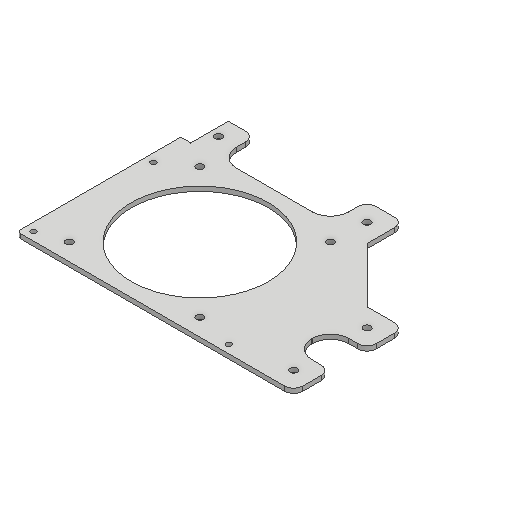
# Autodesk Inventor part: 3DP_PLA_Controller_Case_Top
Saved by Autodesk Inventor 2026.1 (Build 301233000, 233)
## iProperties
Created: 2017-05-26
Part Number: 3DP_PLA_Controller_Case_Top
Material: Ogólny
Document SubType Name: Modeling
Designer: Andrzej
Density: 1 g/cm^3
Appearance: Domyślna
Mass: 20.9942 g
Surface Area: 190.879 cm^2
Volume: 20.9942 cm^3
Author: Andrzej
Autodesk Inventor part; units mm, degrees
ref_plane "YZ Plane" through (0, 0, 0) normal (1, 0, 0) x (0, 1, 0)
ref_plane "XZ Plane" through (0, 0, 0) normal (0, 1, 0) x (-1, 0, 0)
ref_plane "XY Plane" through (0, 0, 0) normal (0, 0, 1) x (1, 0, 0)
sketch "Szkic1" plane through (0, 0, 0) normal (0, 0, 1) x (1, 0, 0)
  line L0 (0, 53.1646) -> (0, 0)
  line L1 (0, 0) -> (98.9175, 0)
  line L2 (98.9175, 0) -> (98.9175, 1.2597)
  line L3 (98.9175, 1.2597) -> (101.455, 3.8466)
  line L4 (101.455, 3.8466) -> (101.455, 38.0126)
  line L5 (101.455, 38.0126) -> (98.9175, 40.5017)
  line L6 (98.9175, 40.5017) -> (98.9175, 50.7051)
  line L7 (98.9175, 50.7051) -> (96.4101, 53.1646)
  line L8 (96.4101, 53.1646) -> (0, 53.1646)
  line L9 (-10, 93.1646) -> (141.455, 93.1646)
  line L10 (141.455, 93.1646) -> (141.455, -17)
  line L11 (141.455, -17) -> (-10, -17)
  line L12 (-10, -17) -> (-10, 93.1646)
  line L13 (91.455, 93.1646) -> (91.455, 43.1646)
  line L14 (91.455, 43.1646) -> (141.455, 43.1646)
  point P0 (-10, 13.9306)
  point P1 (7.9866, -17)
  dimension "d0" = 101.455
  dimension "d1" = 53.1646
  dimension "d2" = 98.9175
  dimension "d21" = 98.9175
  dimension "d22" = 1.2597
  dimension "d23" = 10.2034
  dimension "d24" = 34.166
  dimension "d33" = 40
  dimension "d34" = 40
  dimension "d35" = 17
  dimension "d36" = 10
  dimension "d37" = 50
  dimension "d38" = 50
  constraints: 30 end point, 4 point on line, 2 parallel, 2 perpendicular, 1 horizontal, 1 vertical
  measures "d0" distance between parallel lines of L4 L0
  measures "d1" distance between parallel lines of L1 L8
  measures "d2" distance between parallel lines of L0 L6
  measures "d21" distance between parallel lines of L0 L2
  measures "d22" distance of L2.start L2.end
  measures "d23" distance of L5.end L6.end
  measures "d24" distance of L3.end L5.start
  measures "d33" distance between parallel lines of L10 L4
  measures "d34" distance between parallel lines of L9 L8
  measures "d35" distance between parallel lines of L1 L11
  measures "d36" distance between parallel lines of L12 L0
  measures "d37" distance between parallel lines of L10 L13
  measures "d38" distance between parallel lines of L14 L9
extrude "Wyciągnięcie proste1" add sketch "Szkic1" along normal blind 2.5 contours L8 L13 L14 L6 L5 L4 L3 L2 L1 L0 | L0 L1 L2 L3 L4 L5 L6 L14 L10 L11 L12 L9 L13 L8
sketch "Szkic2" plane through (0, 0, 2.5) normal (0, 0, 1) x (1, 0, 0)
  line L0 (-10, 93.1646) -> (-10, -17) projected
  line L1 (-10, -17) -> (141.455, -17) projected
  line L2 (141.455, -17) -> (141.455, 43.1646) projected
  line L3 (141.455, 43.1646) -> (91.455, 43.1646) projected
  line L4 (91.455, 43.1646) -> (91.455, 93.1646) projected
  line L5 (91.455, 93.1646) -> (-10, 93.1646) projected
  line L6 (10, 93.1646) -> (10, 73.1646)
  line L7 (10, 73.1646) -> (71.455, 73.1646)
  line L8 (71.455, 73.1646) -> (71.455, 93.1646)
  line L9 (91.455, 93.1646) -> (-10, 93.1646) projected
  line L10 (141.455, -17) -> (141.455, 43.1646) projected
  line L11 (141.455, 23.1646) -> (121.455, 23.1646)
  line L12 (121.455, 23.1646) -> (121.455, 3)
  line L13 (121.455, 3) -> (141.455, 3)
  circle A0 centre (45, 28.0823) radius 37.5
  point P0 (0, 0)
  point P1 (131.455, -7)
  point P2 (131.455, 33.1646)
  point P3 (81.455, 83.1646)
  point P4 (0, 83.1646)
  point P5 (9.25, 63.8323)
  point P6 (80.75, 63.8323)
  point P7 (80.75, -7.6677)
  point P8 (9.25, -7.6677)
  dimension "d42" = 20
  dimension "d43" = 20
  dimension "d44" = 20
  dimension "d45" = 20
  dimension "d46" = 20
  dimension "d47" = 20
  dimension "d78" = 10
  dimension "d79" = 10
  dimension "d80" = 10
  dimension "d81" = 10
  dimension "d82" = 10
  dimension "d83" = 10
  dimension "d84" = 10
  dimension "d85" = 10
  dimension "d121" = 75
  dimension "d122" = 35.75
  dimension "d123" = 35.75
  dimension "d124" = 35.75
  dimension "d125" = 35.75
  dimension "d126" = 35.75
  dimension "d127" = 35.75
  dimension "d128" = 35.75
  dimension "d129" = 35.75
  dimension "d139" = 45.0823
  dimension "d140" = 101.455
  dimension "d141" = 90.1646
  dimension "d142" = 55
  constraints: 12 end point, 4 perpendicular, 4 point on line, 1 centre point, 1 horizontal, 1 vertical
  measures "d42" distance between parallel lines of L0 L6
  measures "d43" distance between parallel lines of L4 L8
  measures "d44" distance between parallel lines of L3 L11
  measures "d45" distance between parallel lines of L1 L13
  measures "d46" distance between parallel lines of L5 L7
  measures "d47" distance between parallel lines of L2 L12
  measures "d78" distance from line of L13 point (131.455, -7)
  measures "d79" distance from line of L3 point (131.455, 33.165)
  measures "d80" distance from line of L8 point (81.455, 83.165)
  measures "d81" distance from line of L6 point (0, 83.165)
  measures "d82" distance from line of L2 point (131.455, -7)
  measures "d83" distance from line of L2 point (131.455, 33.165)
  measures "d84" distance from line of L5 point (81.455, 83.165)
  measures "d85" distance from line of L9 point (0, 83.165)
  measures "d121" diameter of A0
  measures "d122" horizontal distance of point (9.25, 63.832) A0.centre
  measures "d123" horizontal distance of A0.centre point (9.25, 63.832)
  measures "d124" horizontal distance of A0.centre point (9.25, -7.668)
  measures "d125" horizontal distance of A0.centre point (9.25, -7.668)
  measures "d126" horizontal distance of point (80.75, 63.832) A0.centre
  measures "d127" horizontal distance of A0.centre point (80.75, 63.832)
  measures "d128" horizontal distance of A0.centre point (80.75, -7.668)
  measures "d129" horizontal distance of A0.centre point (80.75, -7.668)
  measures "d139" distance from line of L7 A0.centre
  measures "d140" distance between parallel lines of L0 L4
  measures "d141" distance between parallel lines of L1 L7
  measures "d142" distance from line of L0 A0.centre
fillet "Zaokrąglenie1" radius 5 4 edges at (-10, 93.1646, 1.25) (91.455, 93.1646, 1.25) (141.455, 43.1646, 1.25) (141.455, -17, 1.25)
hole "Otwór1" at (131.455, -7, 2.5) at (131.455, 33.1646, 2.5) at (81.455, 83.1646, 2.5) at (0, 83.1646, 2.5) direction (0, 0, -1) diameter 4 end through all
fillet "Zaokrąglenie2" radius 2 1 edges at (-10, -17, 1.25)
sketch "Szkic4" plane through (0, 0, 2.5) normal (0, 0, 1) x (1, 0, 0)
  arc A0 (-10, -15) -> (-8, -17) centre (-8, -15) ccw projected
  line L0 (-8, -17) -> (136.455, -17) projected
  arc A1 (136.455, -17) -> (141.455, -12) centre (136.455, -12) ccw projected
  line L1 (141.455, -12) -> (141.455, 38.1646) projected
  arc A2 (141.455, 38.1646) -> (136.455, 43.1646) centre (136.455, 38.1646) ccw projected
  line L2 (136.455, 43.1646) -> (91.455, 43.1646) projected
  line L3 (91.455, 43.1646) -> (91.455, 88.1646) projected
  arc A3 (91.455, 88.1646) -> (86.455, 93.1646) centre (86.455, 88.1646) ccw projected
  line L4 (86.455, 93.1646) -> (-5, 93.1646) projected
  arc A4 (-5, 93.1646) -> (-10, 88.1646) centre (-5, 88.1646) ccw projected
  line L5 (-10, 88.1646) -> (-10, -15) projected
  circle A5 centre (81.455, 83.1646) radius 2 projected
  circle A6 centre (131.455, -7) radius 2 projected
  circle A7 centre (131.455, 33.1646) radius 2 projected
  circle A8 centre (0, 83.1646) radius 2 projected
  point P0 (0, 0)
  point P1 (-5.5, 53.1646)
  point P2 (-5.5, -12.5)
  point P3 (101.455, -12.5)
  dimension "d106" = 40
  dimension "d107" = 4.5
  dimension "d108" = 4.5
  dimension "d109" = 4.5
  dimension "d110" = 4.5
  measures "d106" distance from line of L1 point (101.455, -12.5)
  measures "d107" distance from line of L5 point (-5.5, 53.165)
  measures "d108" distance from line of L0 point (101.455, -12.5)
  measures "d109" distance from line of L0 point (-5.5, -12.5)
  measures "d110" distance from line of L5 point (-5.5, -12.5)
hole "Otwór2" at (-5.5, 53.1646, 2.5) at (-5.5, -12.5, 2.5) at (101.455, -12.5, 2.5) direction (0, 0, -1) diameter 3 end through all
chamfer "Faza2" distance 30 angle 45 1 edges at (91.455, 43.1646, 1.25)
extrude "Wyciągnięcie proste4" cut sketch "Szkic2" against normal through all contours L5 L8 L7 L6 | L13 L12 L11 L2 | A0
hole "Otwór3" at (9.25, 63.8323, 2.5) at (80.75, 63.8323, 2.5) at (80.75, -7.6677, 2.5) at (9.25, -7.6677, 2.5) direction (0, 0, -1) diameter 4 end through all
fillet "Zaokrąglenie3" radius 10 4 edges at (71.455, 73.1646, 1.25) (10, 73.1646, 1.25) (121.455, 23.1646, 1.25) (121.455, 3, 1.25)
fillet "Zaokrąglenie3" radius 5 4 edges at (141.455, 23.1646, 1.25) (141.455, 3, 1.25) (71.455, 93.1646, 1.25) (10, 93.1646, 1.25)
sketch "Szkic7" plane through (0, 0, 2.5) normal (0, 0, 1) x (1, 0, 0)
  arc A0 (10, 88.1646) -> (5, 93.1646) centre (5, 88.1646) ccw projected
  line L0 (5, 93.1646) -> (-5, 93.1646) projected
  arc A1 (-5, 93.1646) -> (-10, 88.1646) centre (-5, 88.1646) ccw projected
  line L1 (-10, 88.1646) -> (-10, -15) projected
  arc A2 (-10, -15) -> (-8, -17) centre (-8, -15) ccw projected
  line L2 (-8, -17) -> (136.455, -17) projected
  arc A3 (136.455, -17) -> (141.455, -12) centre (136.455, -12) ccw projected
  line L3 (141.455, -12) -> (141.455, -2) projected
  arc A4 (141.455, -2) -> (136.455, 3) centre (136.455, -2) ccw projected
  line L4 (136.455, 3) -> (131.455, 3) projected
  arc A5 (121.455, 13) -> (131.455, 3) centre (131.455, 13) ccw projected
  line L5 (121.455, 13) -> (121.455, 13.1646) projected
  arc A6 (131.455, 23.1646) -> (121.455, 13.1646) centre (131.455, 13.1646) ccw projected
  line L6 (131.455, 23.1646) -> (136.455, 23.1646) projected
  arc A7 (136.455, 23.1646) -> (141.455, 28.1646) centre (136.455, 28.1646) ccw projected
  line L7 (141.455, 28.1646) -> (141.455, 38.1646) projected
  arc A8 (141.455, 38.1646) -> (136.455, 43.1646) centre (136.455, 38.1646) ccw projected
  line L8 (136.455, 43.1646) -> (121.455, 43.1646) projected
  line L9 (91.455, 73.1646) -> (121.455, 43.1646) projected
  line L10 (91.455, 73.1646) -> (91.455, 88.1646) projected
  arc A9 (91.455, 88.1646) -> (86.455, 93.1646) centre (86.455, 88.1646) ccw projected
  line L11 (86.455, 93.1646) -> (76.455, 93.1646) projected
  arc A10 (76.455, 93.1646) -> (71.455, 88.1646) centre (76.455, 88.1646) ccw projected
  line L12 (71.455, 88.1646) -> (71.455, 83.1646) projected
  arc A11 (61.455, 73.1646) -> (71.455, 83.1646) centre (61.455, 83.1646) ccw projected
  line L13 (61.455, 73.1646) -> (20, 73.1646) projected
  arc A12 (10, 83.1646) -> (20, 73.1646) centre (20, 83.1646) ccw projected
  line L14 (10, 83.1646) -> (10, 88.1646) projected
  circle A13 centre (80.75, -7.6677) radius 2 projected
  circle A14 centre (9.25, 63.8323) radius 2 projected
  circle A15 centre (80.75, 63.8323) radius 2 projected
  circle A16 centre (9.25, -7.6677) radius 2 projected
  circle A17 centre (45, 28.0823) radius 37.5 projected
  circle A18 centre (-5.5, -12.5) radius 1.5 projected
  circle A19 centre (-5.5, 53.1646) radius 1.5 projected
  circle A20 centre (101.455, -12.5) radius 1.5 projected
  circle A21 centre (0, 83.1646) radius 2 projected
  circle A22 centre (131.455, 33.1646) radius 2 projected
  circle A23 centre (131.455, -7) radius 2 projected
  circle A24 centre (81.455, 83.1646) radius 2 projected
  line L15 (-10, 72.6646) -> (-4.5, 72.6646)
  arc A25 (-5, 93.1646) -> (-10, 88.1646) centre (-5, 88.1646) ccw projected
  line L16 (-4.5, 72.6646) -> (-4.5, 93.1646)
  point P0 (0, 0)
  dimension "d145" = 5.5
  dimension "d147" = 20.5
  constraints: 4 end point, 2 point on line, 1 horizontal, 1 perpendicular
  measures "d145" distance of L15.start L15.end
  measures "d147" distance between parallel lines of L0 L15
extrude "Wyciągnięcie proste5" cut sketch "Szkic7" against normal through all contours L16 L15 L1 A1 L0
equation "\"d47\" = d46"
equation "\"d106\" = d105"
equation "\"d107\" = d110"
equation "\"d108\" = d110"
equation "\"d109\" = d110"
equation "\"d105\" = 40"
